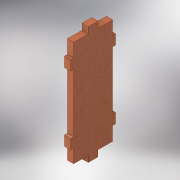
# Autodesk Inventor part: boxSide
Saved by Autodesk Inventor 2017 (Build 210142000, 142)
## iProperties
Created: 2017-05-22
Part Number: boxSide
Material: Generic
Document SubType Name: Modeling
Designer: Dominic Gaiero
Density: 1 g/cm^3
Appearance: Walnut - Natural Polished
Author: Dominic Gaiero
Autodesk Inventor part; units mm, degrees
ref_plane "YZ Plane" through (0, 0, 0) normal (1, 0, 0) x (0, 1, 0)
ref_plane "XZ Plane" through (0, 0, 0) normal (0, 1, 0) x (-1, 0, 0)
ref_plane "XY Plane" through (0, 0, 0) normal (0, 0, 1) x (1, 0, 0)
sketch "Sketch1" plane through (0, 0, 0) normal (1, 0, 0) x (0, 1, 0)
  line L0 (238.1963, 166.0014) -> (238.1963, 162.8264)
  line L1 (238.1963, 162.8264) -> (248.1963, 162.8264)
  line L2 (248.1963, 162.8264) -> (248.1963, 166.0014)
  line L3 (318.1963, 166.0014) -> (318.1963, 162.8264)
  line L4 (318.1963, 162.8264) -> (308.1963, 162.8264)
  line L5 (308.1963, 162.8264) -> (308.1963, 166.0014)
  line L6 (238.1963, 206.0014) -> (238.1963, 209.1764)
  line L7 (238.1963, 209.1764) -> (248.1963, 209.1764)
  line L8 (248.1963, 209.1764) -> (248.1963, 206.0014)
  line L9 (308.1963, 209.1764) -> (308.1963, 206.0014)
  line L10 (318.1963, 209.1764) -> (308.1963, 209.1764)
  line L11 (318.1963, 206.0014) -> (318.1963, 209.1764)
  line L12 (224.1463, 191.0014) -> (217.7963, 191.0014)
  line L13 (217.7963, 191.0014) -> (217.7963, 181.0014)
  line L14 (217.7963, 181.0014) -> (224.1463, 181.0014)
  line L15 (332.2463, 191.0014) -> (338.5963, 191.0014)
  line L16 (338.5963, 191.0014) -> (338.5963, 181.0014)
  line L17 (338.5963, 181.0014) -> (332.2463, 181.0014)
  line L18 (238.1963, 166.0014) -> (224.1463, 166.0014)
  line L19 (332.2463, 166.0014) -> (318.1963, 166.0014)
  line L20 (308.1963, 166.0014) -> (248.1963, 166.0014)
  line L21 (318.1963, 206.0014) -> (332.2463, 206.0014)
  line L22 (224.1463, 206.0014) -> (238.1963, 206.0014)
  line L23 (248.1963, 206.0014) -> (308.1963, 206.0014)
  line L24 (332.2463, 206.0014) -> (332.2463, 191.0014)
  line L25 (332.2463, 181.0014) -> (332.2463, 166.0014)
  line L26 (224.1463, 166.0014) -> (224.1463, 181.0014)
  line L27 (224.1463, 191.0014) -> (224.1463, 206.0014)
  point P0 (0, 0)
  dimension "d22" = 40
  dimension "d23" = 108.1
  dimension "d24" = 14.05
  dimension "d25" = 60
  dimension "d26" = 60
  dimension "d27" = 10
  dimension "d28" = 6.35
  dimension "d29" = 14.05
  dimension "d30" = 14.05
  dimension "d31" = 14.05
  dimension "d32" = 15
  dimension "d33" = 15
  dimension "d34" = 15
  dimension "d35" = 15
  dimension "d36" = 120.8
  dimension "d37" = 3.175
  dimension "d38" = 3.175
  dimension "d39" = 3.175
  dimension "d40" = 40
  dimension "d41" = 46.35
  dimension "d42" = 40
  dimension "d43" = 3.175
  dimension "d44" = 3.175
  dimension "d45" = 3.175
  dimension "d46" = 3.175
  constraints: 56 end point, 17 parallel, 8 perpendicular
  measures "d22" distance of L21.end L19.start
  measures "d23" distance between parallel lines of L25 L26
  measures "d24" distance between parallel lines of L26 L0
  measures "d25" distance between parallel lines of L5 L2
  measures "d26" distance between parallel lines of L9 L8
  measures "d27" distance between parallel lines of L11 L9
  measures "d28" distance between parallel lines of L24 L16
  measures "d29" distance between parallel lines of L24 L11
  measures "d30" distance between parallel lines of L25 L3
  measures "d31" distance between parallel lines of L6 L27
  measures "d32" distance between parallel lines of L18 L14
  measures "d33" distance between parallel lines of L22 L12
  measures "d34" distance between parallel lines of L17 L19
  measures "d35" distance between parallel lines of L21 L15
  measures "d36" distance between parallel lines of L16 L13
  measures "d37" distance between parallel lines of L22 L7
  measures "d38" distance between parallel lines of L23 L10
  measures "d39" distance between parallel lines of L20 L4
  measures "d40" distance between parallel lines of L23 L20
  measures "d41" distance between parallel lines of L10 L4
  measures "d42" distance between parallel lines of L18 L22
  measures "d43" distance between parallel lines of L18 L1
  measures "d44" distance between parallel lines of L7 L23
  measures "d45" distance between parallel lines of L10 L21
  measures "d46" distance between parallel lines of L20 L1
extrude "Extrusion1" add sketch "Sketch1" along normal blind 6.35
body "Solid1"
